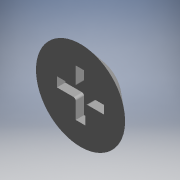
# Autodesk Inventor part: 3628_
Saved by Autodesk Inventor 2017.3 (Build 213256000, 256)
## iProperties
Part Number: 3628_
Material: Generic
Catalog Web Link: www.cadenas.de
Description: 3265, 3268-Countersunk Bolt
Vendor: 8020
Document SubType Name: Modeling
Designer: partserver
Manufacturer: 8020
Mass: 0.0812868 g
Surface Area: 1.86203 cm^2
Volume: 0.0812868 cm^3
Density: 1 g/cm^3
Appearance: PSOLRGB-192-192-192
Category: PARTsolutions
Company: 8020
Title: 3628_
Author: Cadenas PARTsolutions
Comments: Countersunk Bolt
PSOL_IDENT_0: {$CADENAS_DATA\23d-libs\8020\inch\linear_motion\csunk_bolt.prj},154 {VTYP=3D},{NB=3628_},{LINA=3628_
PSOL_IDENT_1: },{NN=3265, 3268},{DATE=31.07.2020 09:21:20},{GEOMDATE=15.06.2012 00:00:00},{VERSION=},{LINEID=50},{
PSOL_IDENT_2: WBVAR=},{WBNUMERIC=}  {NB=3628_},{LINA=3628_},{KT=DUMMY},{PN=3628},{PN1=10-24},{A=1.500},{TH=0.250},
PSOL_IDENT_3: {CS=0.385},{HD1=0.201}
NB: 3628_
NN: 3265, 3268
NT: Countersunk Bolt
NBSYN: $PN._
LINA: 3628_
CATALOG: 80/20
PN: 3628
PN1: 10-24
A: 1.5
TH: 0.25
CS: 0.385
HD1: 0.201
SUPPLIER: 8020
ARTICLENO: 3628_
BOMINFO: 3628_
CREATOR: CADENAS GmbH
Autodesk Inventor part; units mm, degrees
sketch "Sketch_3" plane through (0, 0, 0) normal (0, 0, 1) x (1, 0, 0)
  line L0 (0, -1.9608) -> (0, 0.1172)
  line L1 (0, 0.1172) -> (2.413, 0.1172)
  line L2 (2.413, 0.1172) -> (4.8895, -1.9608)
  line L3 (4.8895, -1.9608) -> (0, -1.9608)
  line L4 (0, -1.9608) -> (0, 0.1172)
  constraints: 10 end point
revolve "Revolution1" add sketch "Sketch_3" angle 360 about axis through (0, -1.9608, 0) along (0, -1, 0)
sketch "Sketch_4" plane through (0, -1.9608, 0) normal (0, -1, 0) x (1, 0, 0)
  line L0 (-2.5883, 0.5283) -> (-2.5883, -0.5283)
  line L1 (-2.5883, -0.5283) -> (-0.7823, -0.5283)
  arc A0 (-0.5283, -0.7823) -> (-0.7823, -0.5283) centre (-0.7823, -0.7823) ccw
  line L2 (-0.5283, -0.7823) -> (-0.5283, -2.5883)
  line L3 (-0.5283, -2.5883) -> (0.5283, -2.5883)
  line L4 (0.5283, -2.5883) -> (0.5283, -0.7823)
  arc A1 (0.7823, -0.5283) -> (0.5283, -0.7823) centre (0.7823, -0.7823) ccw
  line L5 (0.7823, -0.5283) -> (2.5883, -0.5283)
  line L6 (2.5883, -0.5283) -> (2.5883, 0.5283)
  line L7 (2.5883, 0.5283) -> (0.7823, 0.5283)
  arc A2 (0.5283, 0.7823) -> (0.7823, 0.5283) centre (0.7823, 0.7823) ccw
  line L8 (0.5283, 0.7823) -> (0.5283, 2.5883)
  line L9 (0.5283, 2.5883) -> (-0.5283, 2.5883)
  line L10 (-0.5283, 2.5883) -> (-0.5283, 0.7823)
  arc A3 (-0.7823, 0.5283) -> (-0.5283, 0.7823) centre (-0.7823, 0.7823) ccw
  line L11 (-0.7823, 0.5283) -> (-2.5883, 0.5283)
  constraints: 24 end point, 8 point on circle, 4 centre point
extrude "Extrusion1" cut sketch "Sketch_4" against normal blind 0.9195
ref_plane "screw_XY" through (0, 0, 0) normal (0, 1, 0) x (1, 0, 0)
ref_plane "screw_YZ" through (0, 0, 0) normal (1, 0, 0) x (0, 0, -1)
ref_plane "screw_ZX" through (0, 0, 0) normal (0, 0, -1) x (0, 1, 0)
body "Solid1"
